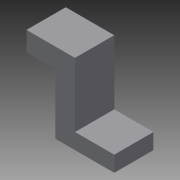
# Autodesk Inventor part: potentiometer stand
Saved by Autodesk Inventor 2015 (Build 190159000, 159)
## iProperties
Created: 2015-02-22
Part Number: potentiometer stand
Material: Generic
Document SubType Name: Modeling
Designer: szymsea16
Density: 1 g/cm^3
Appearance: Default
Author: szymsea16
Autodesk Inventor part; units mm, degrees
ref_plane "YZ Plane" through (0, 0, 0) normal (1, 0, 0) x (0, 1, 0)
ref_plane "XZ Plane" through (0, 0, 0) normal (0, 1, 0) x (-1, 0, 0)
ref_plane "XY Plane" through (0, 0, 0) normal (0, 0, 1) x (1, 0, 0)
sketch "Sketch1" plane through (0, 0, 0) normal (0, 0, 1) x (1, 0, 0)
  line L0 (0, 0) -> (6.35, 0)
  line L1 (6.35, 0) -> (6.35, 19.5072)
  line L2 (6.35, 19.5072) -> (0, 19.5072)
  line L3 (0, 19.5072) -> (0, 0)
  line L4 (0, 0) -> (6.35, 0)
  line L5 (6.35, 0) -> (6.35, 10.0076)
  line L6 (6.35, 10.0076) -> (0, 10.0076)
  line L7 (0, 10.0076) -> (0, 0)
  line L8 (6.35, 19.5072) -> (-9.3472, 19.5072)
  line L9 (-9.3472, 19.5072) -> (-9.3472, 25.8572)
  line L10 (-9.3472, 25.8572) -> (6.35, 25.8572)
  line L11 (6.35, 25.8572) -> (6.35, 19.5072)
  line L12 (6.35, 0) -> (19.05, 0)
  line L13 (19.05, 0) -> (19.05, 5.08)
  line L14 (19.05, 5.08) -> (6.35, 5.08)
  line L15 (6.35, 5.08) -> (6.35, 0)
  dimension "d0" = 6.35
  dimension "d1" = 19.5072
  dimension "d2" = 10.0076
  dimension "d3" = 15.6972
  dimension "d4" = 6.35
  dimension "d5" = 12.7
  dimension "d6" = 5.08
  constraints: 32 end point, 8 parallel, 4 horizontal, 4 perpendicular, 1 point on line
  measures "d0" distance of L2.end L1.end
  measures "d1" distance of L1.end L0.end
  measures "d2" distance of L5.end L4.end
  measures "d3" distance of L9.end L10.end
  measures "d4" distance of L8.end L9.end
  measures "d5" distance of L14.end L13.end
  measures "d6" distance of L13.end L12.end
extrude "Extrusion1" add sketch "Sketch1" along normal blind 12.7
body "Solid1"
